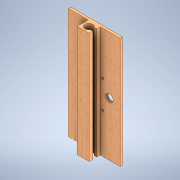
# Autodesk Inventor part: Rack Base
Saved by Autodesk Inventor 2020 (Build 240168000, 168)
## iProperties
Created: 2021-06-18
Part Number: Rack Base
Material: Generic
Document SubType Name: Modeling
Designer: ugwue
Density: 1 g/cm^3
Appearance: Cherry - Natural Low Gloss
Author: ugwue
Autodesk Inventor part; units mm, degrees
ref_plane "YZ Plane" through (0, 0, 0) normal (1, 0, 0) x (0, 1, 0)
ref_plane "XZ Plane" through (0, 0, 0) normal (0, 1, 0) x (-1, 0, 0)
ref_plane "XY Plane" through (0, 0, 0) normal (0, 0, 1) x (1, 0, 0)
sketch "Sketch1" plane through (0, 0, 0) normal (0, 0, 1) x (1, 0, 0)
  line L0 (0, 0) -> (60, 0)
  line L1 (60, 0) -> (60, 140)
  line L2 (60, 140) -> (0, 140)
  line L3 (0, 140) -> (0, 0)
  dimension "d0" = 60
  dimension "d1" = 140
  constraints: 8 end point, 2 parallel, 1 horizontal, 1 perpendicular
  measures "d0" distance of L2.end L1.end
  measures "d1" distance of L1.end L0.end
extrude "Extrusion1" add sketch "Sketch1" along normal blind 3
sketch "Sketch4" plane through (0, 0, 3) normal (0, 0, 1) x (1, 0, 0)
  point P0 (0, 0)
sketch "Sketch5" plane through (0, 0, 3) normal (0, 0, 1) x (1, 0, 0)
  circle A0 centre (38.0013, 85.4781) radius 1.5
  circle A1 centre (38.0013, 50.4781) radius 1.5
  line L0 (60, 0) -> (60, 140) projected
  circle A2 centre (46.5013, 67.9781) radius 4.75
  line L1 (60, 0) -> (60, 140) projected
  line L2 (60, 67.9781) -> (70, 67.9781) construction
  point P0 (0, 0)
  dimension "d11" = 3
  constraints: 3 centre point, 2 end point, 1 horizontal, 1 point on line
  measures "d11" diameter of A0
extrude "Extrusion4" cut sketch "Sketch5" against normal blind 145
sketch "Sketch6" plane through (0, 0, 0) normal (-1, 0, 0) x (0, 0, 1)
  line L0 (0, 140) -> (0, 0) projected
  line L1 (3, 0) -> (3, 140) projected
  line L2 (0, 0) -> (3, 0)
  line L3 (3, 0) -> (3, 140)
  line L4 (3, 140) -> (0, 140)
  line L5 (0, 140) -> (0, 0)
  constraints: 8 end point, 2 parallel, 1 horizontal, 1 perpendicular
extrude "Extrusion5" add sketch "Sketch6" along normal blind 5
sketch "Sketch7" plane through (60, 140, 3) normal (0, 1, 0) x (1, 0, 0)
  line L0 (-65, 0) -> (-65, 3) projected
  line L1 (-65, 3) -> (0, 3)
  line L2 (0, 3) -> (0, -17)
  line L3 (0, -17) -> (-65, -17)
  line L4 (-65, -17) -> (-65, 3)
  arc A0 (-28.1699, -4.5) -> (-28.1699, -9.5) centre (-32.5, -7) ccw
  line L5 (-25, -9.5) -> (-25, -4.5)
  line L6 (-40, -4.5) -> (-25, -9.5) construction
  line L7 (-40, -9.5) -> (-25, -4.5) construction
  line L8 (-28.1699, -9.5) -> (-25, -9.5)
  line L9 (-25, -4.5) -> (-28.1699, -4.5)
  point P0 (-60, 3)
  dimension "d18" = 65
  dimension "d19" = 20
  constraints: 18 end point, 3 parallel, 2 midpoint, 2 point on circle, 1 centre point, 1 horizontal, 1 perpendicular
  measures "d18" distance of L2.end L3.end
  measures "d19" distance of L1.end L2.end
sketch "Sketch8" plane through (0, 0, 3) normal (0, 0, 1) x (1, 0, 0)
  line L0 (35, 0) -> (35, 140)
  line L1 (35, 140) -> (20, 140)
  line L2 (20, 140) -> (20, 0)
  line L3 (20, 0) -> (35, 0)
  line L4 (35, 0) -> (20, 140) construction
  line L5 (35, 140) -> (20, 0) construction
  line L6 (60, 0) -> (60, 140) projected
  line L7 (35, 0) -> (175, 0) construction
  point P0 (0, 0)
  point P1 (27.5, 70)
  dimension "d21" = 140
  dimension "d22" = 90
  dimension "d23" = 15
  constraints: 14 end point, 3 parallel, 2 midpoint, 2 perpendicular, 1 horizontal
  measures "d21" distance of L0.start L0.end
  measures "d22" angle of L7 L0
  measures "d23" distance of L1.end L0.end
extrude "Extrusion6" add sketch "Sketch8" along normal blind 14
extrude "Extrusion7" cut sketch "Sketch7" against normal blind 140 contours L9 L5 L8 A0
sketch "Sketch9" plane through (0, 0, 3) normal (0, 0, 1) x (1, 0, 0)
  point P0 (0, 0)
body "Solid1"
